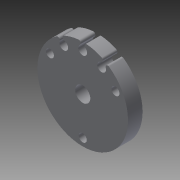
# Autodesk Inventor part: UpperPlate
Saved by Autodesk Inventor 2014 SP1 (Build 180222100, 222)
## iProperties
Created: 2013-12-26
Part Number: UpperPlate
Material: Generic
Document SubType Name: Modeling
Designer: Jack
Density: 1 g/cm^3
Appearance: Default
Author: Jack
Autodesk Inventor part; units mm, degrees
ref_plane "YZ Plane" through (0, 0, 0) normal (1, 0, 0) x (0, 1, 0)
ref_plane "XZ Plane" through (0, 0, 0) normal (0, 1, 0) x (-1, 0, 0)
ref_plane "XY Plane" through (0, 0, 0) normal (0, 0, 1) x (1, 0, 0)
sketch "Sketch1" plane through (0, 0, 0) normal (0, 1, 0) x (-1, 0, 0)
  circle A0 centre (0, 0) radius 16.5 construction
  circle A1 centre (0, 0) radius 3.3
  arc A2 (-0.8286, 18.2098) -> (0.8286, 18.2098) centre (0, 16.5) ccw
  line L0 (0, 0) -> (9.875, 17.104) construction
  line L1 (0, 0) -> (-9.875, 17.104) construction
  line L2 (0, 0) -> (-17.104, 9.875) construction
  line L3 (0, 0) -> (17.104, 9.875) construction
  line L4 (-19.75, 0) -> (19.75, 0) construction
  circle A3 centre (0, -16.5) radius 1.75
  circle A4 centre (14.2894, 8.25) radius 1.75
  circle A5 centre (-14.2894, 8.25) radius 1.75
  arc A6 (8.3873, 16.1844) -> (9.8225, 15.3559) centre (8.25, 14.2894) ccw
  arc A7 (-9.8225, 15.3559) -> (-8.3873, 16.1844) centre (-8.25, 14.2894) ccw
  line L5 (0, 0) -> (0.75, 16.4829) construction
  line L6 (-0.75, 16.4829) -> (0, 0) construction
  line L7 (-7.592, 14.6496) -> (0, 0) construction
  line L8 (-8.891, 13.8996) -> (0, 0) construction
  line L9 (7.592, 14.6496) -> (0, 0) construction
  line L10 (8.891, 13.8996) -> (0, 0) construction
  line L11 (-8.3873, 16.1844) -> (-9.0873, 17.5352)
  line L12 (-9.8225, 15.3559) -> (-10.6422, 16.6375)
  line L13 (-0.8286, 18.2098) -> (-0.8977, 19.7296)
  line L14 (0.8286, 18.2098) -> (0.8977, 19.7296)
  line L15 (8.3873, 16.1844) -> (9.0873, 17.5352)
  line L16 (9.8225, 15.3559) -> (10.6422, 16.6375)
  arc A8 (9.0873, 17.5352) -> (0.8977, 19.7296) centre (0, 0) ccw
  arc A9 (-0.8977, 19.7296) -> (-9.0873, 17.5352) centre (0, 0) ccw
  arc A10 (-10.6422, 16.6375) -> (10.6422, 16.6375) centre (0, 0) ccw
  dimension "d1" = 33
  dimension "d2" = 6.6
  dimension "d3" = 3.8
  dimension "d4" = 30
  dimension "d5" = 60
  dimension "d6" = 60
  dimension "d7" = 30
  dimension "d8" = 3.5
  dimension "d9" = 3.5
  dimension "d10" = 3.5
  dimension "d11" = 3.8
  dimension "d12" = 3.8
  dimension "d13" = 0.75
  dimension "d14" = 0.75
  dimension "d15" = 0.75
  dimension "d16" = 0.75
  dimension "d17" = 0.75
  dimension "d18" = 0.75
  dimension "d20" = 19.75
  dimension "d21" = 19.75
  dimension "d22" = 19.75
  constraints: 34 end point, 16 point on circle, 12 collinear, 10 centre point, 5 point on line, 3 coincident, 2 horizontal, 2 midpoint, 2 vertical alignment, 14 other
  measures "d2" diameter of A1
  measures "d3" diameter of A2
  measures "d4" angle of L4 L3
  measures "d5" angle of L4 L0
  measures "d6" angle of L4 L1
  measures "d7" angle of L4 L2
  measures "d8" diameter of A3
  measures "d9" diameter of A4
  measures "d10" diameter of A5
  measures "d11" diameter of A6
  measures "d12" diameter of A7
  measures "d13" distance from line of L1 L8.start
  measures "d14" distance from line of L1 L7.start
  measures "d15" horizontal distance of A2.centre L6.start
  measures "d16" horizontal distance of A2.centre L5.end
  measures "d17" distance from line of L0 L10.start
  measures "d18" distance from line of L0 L9.start
  measures "d20" radius of A9
  measures "d21" radius of A8
  measures "d22" radius of A10
extrude "Extrusion1" add sketch "Sketch1" along normal blind 6.35
fillet "Fillet1" radius 0.9 6 edges at (9.0873, 3.175, 17.5352) (10.6422, 3.175, 16.6375) (-0.8977, 3.175, 19.7296) (0.8977, 3.175, 19.7296) (-10.6422, 3.175, 16.6375) (-9.0873, 3.175, 17.5352)
fillet "Fillet2" radius 0.9 6 edges at (-9.8225, 3.175, 15.3559) (-0.8286, 3.175, 18.2098) (-8.3873, 3.175, 16.1844) (0.8286, 3.175, 18.2098) (8.3873, 3.175, 16.1844) (9.8225, 3.175, 15.3559)
body "Solid1"
